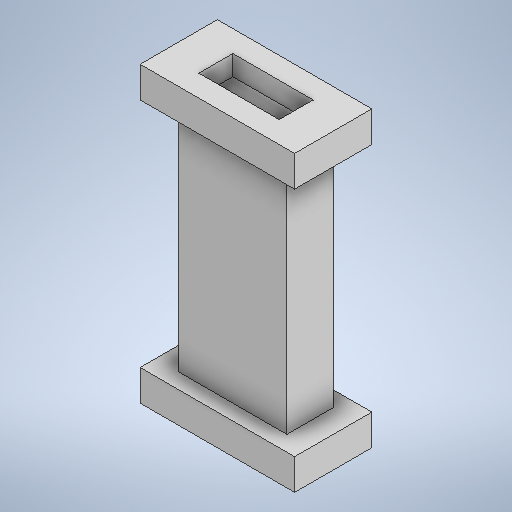
# Autodesk Inventor part: 差分線圈感應
Saved by Autodesk Inventor 2025.2 (Build 292293000, 293)
## iProperties
Created: 2025-07-14
Part Number: 差分線圈感應
Material: 一般
Document SubType Name: Modeling
Designer: 123
Density: 1 g/cm^3
Appearance: 預設
Author: 123
Autodesk Inventor part; units mm, degrees
ref_plane "YZ Plane" through (0, 0, 0) normal (1, 0, 0) x (0, 1, 0)
ref_plane "XZ Plane" through (0, 0, 0) normal (0, 1, 0) x (-1, 0, 0)
ref_plane "XY Plane" through (0, 0, 0) normal (0, 0, 1) x (1, 0, 0)
sketch "草圖7" plane through (0, 0, 0) normal (0, 1, 0) x (-1, 0, 0)
  line L0 (5, 2.5) -> (-5, 2.5)
  line L1 (-5, 2.5) -> (-5, -2.5)
  line L2 (-5, -2.5) -> (5, -2.5)
  line L3 (5, -2.5) -> (5, 2.5)
  line L4 (5, 2.5) -> (-5, -2.5) construction
  line L5 (-5, 2.5) -> (5, -2.5) construction
  line L6 (2.6, 1.1) -> (-2.6, 1.1)
  line L7 (-2.6, 1.1) -> (-2.6, -1.1)
  line L8 (-2.6, -1.1) -> (2.6, -1.1)
  line L9 (2.6, -1.1) -> (2.6, 1.1)
  line L10 (2.6, 1.1) -> (-2.6, -1.1) construction
  line L11 (-2.6, 1.1) -> (2.6, -1.1) construction
  point P0 (0, 0)
  dimension "d18" = 10
  dimension "d19" = 5
  dimension "d20" = 2.2
  dimension "d21" = 5.2
  constraints: 24 end point, 4 midpoint, 4 parallel, 2 horizontal, 2 perpendicular
  measures "d18" distance of L1.end L2.end
  measures "d19" distance of L2.end L0.start
  measures "d20" distance of L8.end L6.start
  measures "d21" distance of L7.end L8.end
extrude "擠出7" add sketch "草圖7" against normal blind 2
sketch "草圖8" plane through (0, 0, 0) normal (0, 1, 0) x (1, 0, 0)
  line L0 (-3.5, -1.5) -> (3.5, -1.5)
  line L1 (3.5, -1.5) -> (3.5, 1.5)
  line L2 (3.5, 1.5) -> (-3.5, 1.5)
  line L3 (-3.5, 1.5) -> (-3.5, -1.5)
  line L4 (-3.5, -1.5) -> (3.5, 1.5) construction
  line L5 (3.5, -1.5) -> (-3.5, 1.5) construction
  point P0 (0, 0)
  dimension "d24" = 7
  dimension "d25" = 3
  constraints: 12 end point, 2 midpoint, 2 parallel, 1 horizontal, 1 perpendicular
  measures "d24" distance of L1.end L2.end
  measures "d25" distance of L2.end L0.start
extrude "擠出8" add sketch "草圖8" along normal blind 15
sketch "草圖9" plane through (0, 15, 0) normal (0, 1, 0) x (1, 0, 0)
  line L0 (5, -2.5) -> (5, 2.5) projected
  line L1 (-5, -2.5) -> (5, -2.5)
  line L2 (5, -2.5) -> (5, 2.5)
  line L3 (5, 2.5) -> (-5, 2.5)
  line L4 (-5, 2.5) -> (-5, -2.5)
  line L5 (-5, -2.5) -> (5, 2.5) construction
  line L6 (5, -2.5) -> (-5, 2.5) construction
  point P0 (0, 0)
  constraints: 12 end point, 2 midpoint, 2 parallel, 1 horizontal, 1 perpendicular
extrude "擠出9" add sketch "草圖9" along normal blind 2
sketch "草圖10" plane through (0, 17, 0) normal (0, 1, 0) x (1, 0, 0)
  line L0 (-2.6, 1.1) -> (2.6, 1.1) projected
  line L1 (-2.6, -1.1) -> (2.6, -1.1)
  line L2 (2.6, -1.1) -> (2.6, 1.1)
  line L3 (2.6, 1.1) -> (-2.6, 1.1)
  line L4 (-2.6, 1.1) -> (-2.6, -1.1)
  line L5 (-2.6, -1.1) -> (2.6, 1.1) construction
  line L6 (2.6, -1.1) -> (-2.6, 1.1) construction
  point P0 (0, 0)
  constraints: 12 end point, 2 midpoint, 2 parallel, 1 horizontal, 1 perpendicular
extrude "擠出10" cut sketch "草圖10" against normal blind 1.3
